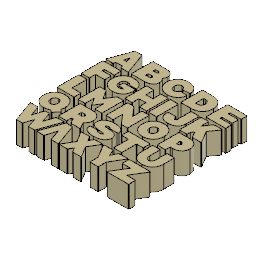
AlphaBlocks (Autodesk Fusion 360 design; units mm, degrees)
Autodesk Fusion 360 part; units mm, degrees
sketch "Sketch1" plane through (0, 0, 0) normal (0, 1, 0) x (1, 0, 0)
  arc A0 (47.4557, -43.7833) -> (46.9512, -43.2752) centre (47.4934, -43.2413) cw
  line L0 (46.9512, -43.2752) -> (46.9512, -18.8912)
  arc A1 (46.9512, -18.8912) -> (47.4557, -18.3833) centre (47.4934, -18.9252) cw
  line L1 (47.4557, -18.3833) -> (62.4769, -18.3833)
  spline S0 degree 3 poles (62.4769, -18.3833) (68.3824, -18.3833) (71.5045, -21.6429) (71.5045, -25.5799) knots 0 0 0 0 1 1 1 1
  arc A2 (71.5045, -25.5799) -> (69.5643, -30.1096) centre (65.5084, -25.6919) cw
  line L2 (69.5643, -30.1096) -> (69.5643, -30.1519)
  arc A3 (69.5643, -30.1519) -> (72.3512, -35.8669) centre (65.3567, -35.7408) cw
  spline S1 degree 3 poles (72.3512, -35.8669) (72.3512, -40.7353) (68.7211, -43.7833) (62.3923, -43.7833) knots 0 0 0 0 1 1 1 1
  line L3 (62.3923, -43.7833) -> (47.4557, -43.7833)
  line L4 (56.5679, -27.9083) -> (60.198, -27.9083)
  spline S2 degree 3 poles (60.198, -27.9083) (61.4645, -27.9083) (61.8843, -27.3579) (61.8843, -26.6383) knots 0 0 0 0 1 1 1 1
  spline S3 degree 3 poles (61.8843, -26.6383) (61.8843, -25.9186) (61.3798, -25.3683) (59.9863, -25.3683) knots 0 0 0 0 1 1 1 1
  line L5 (59.9863, -25.3683) -> (56.5679, -25.3683)
  line L6 (56.5679, -25.3683) -> (56.5679, -27.9083)
  line L7 (56.5679, -36.5866) -> (60.4943, -36.5866)
  spline S4 degree 3 poles (60.4943, -36.5866) (62.0536, -36.5866) (62.7309, -36.0786) (62.7309, -35.1472) knots 0 0 0 0 1 1 1 1
  spline S5 degree 3 poles (62.7309, -35.1472) (62.7309, -34.2159) (62.0536, -33.6232) (60.4943, -33.6232) knots 0 0 0 0 1 1 1 1
  line L8 (60.4943, -33.6232) -> (56.5679, -33.6232)
  line L9 (56.5679, -33.6232) -> (56.5679, -36.5866)
  spline S6 degree 3 poles (93.0698, -29.651) (92.7171, -29.651) (92.4913, -29.404) (92.3643, -28.9948) knots 0 0 0 0 1 1 1 1
  spline S7 degree 3 poles (92.3643, -28.9948) (91.8245, -27.111) (90.5545, -26.1726) (88.6636, -26.1726) knots 0 0 0 0 1 1 1 1
  spline S8 degree 3 poles (88.6636, -26.1726) (86.5823, -26.1726) (84.5397, -27.9753) (84.5397, -31.0868) knots 0 0 0 0 1 1 1 1
  spline S9 degree 3 poles (84.5397, -31.0868) (84.5397, -34.1171) (86.4694, -35.9622) (88.6636, -35.9622) knots 0 0 0 0 1 1 1 1
  spline S10 degree 3 poles (88.6636, -35.9622) (90.4275, -35.9622) (91.7469, -35.1014) (92.3643, -33.3798) knots 0 0 0 0 1 1 1 1
  arc A4 (92.3643, -33.3798) -> (93.1757, -32.7272) centre (93.1658, -33.5456) cw
  line L10 (93.1757, -32.7272) -> (100.4217, -32.7272)
  arc A5 (100.4217, -32.7272) -> (101.152, -33.4645) centre (100.3801, -33.4987) cw
  spline S11 degree 3 poles (101.152, -33.4645) (101.152, -39.5676) (95.7192, -43.7868) (88.6636, -43.7868) knots 0 0 0 0 1 1 1 1
  spline S12 degree 3 poles (88.6636, -43.7868) (81.4564, -43.7868) (75.752, -38.6256) (75.752, -31.0868) knots 0 0 0 0 1 1 1 1
  spline S13 degree 3 poles (75.752, -31.0868) (75.752, -23.5479) (81.4564, -18.3868) (88.6636, -18.3868) knots 0 0 0 0 1 1 1 1
  spline S14 degree 3 poles (88.6636, -18.3868) (95.9873, -18.3868) (101.152, -23.0576) (101.152, -28.8325) knots 0 0 0 0 1 1 1 1
  spline S15 degree 3 poles (101.152, -28.8325) (101.152, -29.2841) (100.9227, -29.6545) (100.4958, -29.6545) knots 0 0 0 0 1 1 1 1
  line L11 (100.4958, -29.6545) -> (93.0698, -29.651)
  arc A6 (105.0643, -43.7833) -> (104.5774, -43.2752) centre (105.113, -43.2492) cw
  line L12 (104.5774, -43.2752) -> (104.5774, -18.8912)
  arc A7 (104.5774, -18.8912) -> (105.0643, -18.3833) centre (105.113, -18.9173) cw
  line L13 (105.0643, -18.3833) -> (115.951, -18.3833)
  spline S16 degree 3 poles (115.951, -18.3833) (124.2695, -18.3833) (129.9774, -23.3786) (129.9774, -31.0833) knots 0 0 0 0 1 1 1 1
  spline S17 degree 3 poles (129.9774, -31.0833) (129.9774, -38.6609) (125.1656, -43.7833) (116.0321, -43.7833) knots 0 0 0 0 1 1 1 1
  line L14 (116.0321, -43.7833) -> (105.0643, -43.7833)
  line L15 (113.8837, -26.4266) -> (113.8837, -35.7399)
  line L16 (113.8837, -35.7399) -> (116.0004, -35.7399)
  spline S18 degree 3 poles (116.0004, -35.7399) (119.1401, -35.7399) (120.6888, -33.976) (120.6888, -31.0833) knots 0 0 0 0 1 1 1 1
  spline S19 degree 3 poles (120.6888, -31.0833) (120.6888, -28.1199) (118.8544, -26.4266) (115.9581, -26.4266) knots 0 0 0 0 1 1 1 1
  line L17 (115.9581, -26.4266) -> (113.8837, -26.4266)
  line L18 (143.5806, -34.6816) -> (143.5806, -36.5866)
  line L19 (143.5806, -36.5866) -> (156.3088, -36.5866)
  arc A8 (156.3088, -36.5866) -> (156.9014, -37.1792) centre (156.2038, -37.2843) cw
  line L20 (156.9014, -37.1792) -> (156.9014, -43.1765)
  arc A9 (156.9014, -43.1765) -> (156.3088, -43.7691) centre (156.2038, -43.0714) cw
  line L21 (156.3088, -43.7691) -> (134.4083, -43.7691)
  arc A10 (134.4083, -43.7691) -> (133.8968, -43.2611) centre (134.4423, -43.2234) cw
  line L22 (133.8968, -43.2611) -> (133.8968, -18.8912)
  arc A11 (133.8968, -18.8912) -> (134.4083, -18.3833) centre (134.4423, -18.929) cw
  line L23 (134.4083, -18.3833) -> (156.2982, -18.3833)
  arc A12 (156.2982, -18.3833) -> (156.8909, -18.9759) centre (156.1932, -19.0809) cw
  line L24 (156.8909, -18.9759) -> (156.8909, -24.9731)
  arc A13 (156.8909, -24.9731) -> (156.2982, -25.5658) centre (156.1932, -24.8681) cw
  line L25 (156.2982, -25.5658) -> (143.5806, -25.5658)
  line L26 (143.5806, -25.5658) -> (143.5806, -27.4708)
  line L27 (143.5806, -27.4708) -> (155.0353, -27.4708)
  arc A14 (155.0353, -27.4708) -> (155.6279, -28.0635) centre (154.9302, -28.1685) cw
  line L28 (155.6279, -28.0635) -> (155.6279, -34.0607)
  arc A15 (155.6279, -34.0607) -> (155.0353, -34.6534) centre (154.9302, -33.9557) cw
  line L29 (155.0353, -34.6534) -> (143.5806, -34.6816)
  arc A16 (17.6389, -72.2207) -> (17.1309, -71.7127) centre (17.6764, -71.6751) cw
  line L30 (17.1309, -71.7127) -> (17.1309, -47.3287)
  arc A17 (17.1309, -47.3287) -> (17.6389, -46.8207) centre (17.6764, -47.3662) cw
  line L31 (17.6389, -46.8207) -> (37.8319, -46.8207)
  arc A18 (37.8319, -46.8207) -> (38.4281, -47.4133) centre (37.7305, -47.5189) cw
  line L32 (38.4281, -47.4133) -> (38.4281, -54.2713)
  arc A19 (38.4281, -54.2713) -> (37.8319, -54.864) centre (37.7305, -54.1658) cw
  line L33 (37.8319, -54.864) -> (26.8111, -54.864)
  line L34 (26.8111, -54.864) -> (26.8111, -57.404)
  line L35 (26.8111, -57.404) -> (36.9923, -57.404)
  arc A20 (36.9923, -57.404) -> (37.5849, -57.9967) centre (36.8873, -58.1017) cw
  line L36 (37.5849, -57.9967) -> (37.5849, -64.4313)
  arc A21 (37.5849, -64.4313) -> (36.9923, -65.024) centre (36.8873, -64.3263) cw
  line L37 (36.9923, -65.024) -> (26.8111, -65.024)
  line L38 (26.8111, -65.024) -> (26.8111, -71.7268)
  arc A22 (26.8111, -71.7268) -> (26.2996, -72.2348) centre (26.2656, -71.689) cw
  line L39 (26.2996, -72.2348) -> (17.6389, -72.2207)
  arc A23 (83.4743, -119.9444) -> (84.7619, -120.6817) centre (83.5073, -121.3799) cw
  spline S20 degree 3 poles (84.7619, -120.6817) (85.217, -121.3379) (86.2154, -121.8283) (88.2474, -121.8283) knots 0 0 0 0 1 1 1 1
  spline S21 degree 3 poles (88.2474, -121.8283) (90.4064, -121.8283) (91.1542, -121.1227) (91.1542, -120.5195) knots 0 0 0 0 1 1 1 1
  spline S22 degree 3 poles (91.1542, -120.5195) (91.1542, -120.0679) (90.738, -119.8139) (89.535, -119.6975) knots 0 0 0 0 1 1 1 1
  line L40 (89.535, -119.6975) -> (83.7247, -119.126)
  spline S23 degree 3 poles (83.7247, -119.126) (78.6201, -118.6321) (75.2157, -116.5049) (75.2157, -112.3245) knots 0 0 0 0 1 1 1 1
  spline S24 degree 3 poles (75.2157, -112.3245) (75.2157, -106.9975) (79.9465, -103.2298) (87.4607, -103.2298) knots 0 0 0 0 1 1 1 1
  spline S25 degree 3 poles (87.4607, -103.2298) (95.5534, -103.2298) (99.1623, -106.7576) (99.1623, -110.1125) knots 0 0 0 0 1 1 1 1
  arc A24 (99.1623, -110.1125) -> (98.044, -111.3402) centre (97.9705, -110.1501) cw
  line L41 (98.044, -111.3402) -> (90.6956, -111.3402)
  arc A25 (90.6956, -111.3402) -> (89.7431, -110.8922) centre (90.6223, -110.2597) cw
  spline S26 degree 3 poles (89.7431, -110.8922) (89.3692, -110.4406) (88.706, -109.9467) (87.4183, -109.9467) knots 0 0 0 0 1 1 1 1
  spline S27 degree 3 poles (87.4183, -109.9467) (85.3828, -109.9467) (84.6772, -110.7264) (84.6772, -111.3014) knots 0 0 0 0 1 1 1 1
  spline S28 degree 3 poles (84.6772, -111.3014) (84.6772, -111.6542) (85.0124, -111.9541) (86.0072, -112.0387) knots 0 0 0 0 1 1 1 1
  line L42 (86.0072, -112.0387) -> (91.694, -112.5714)
  spline S29 degree 3 poles (91.694, -112.5714) (98.1675, -113.1852) (100.6158, -116.011) (100.6158, -119.821) knots 0 0 0 0 1 1 1 1
  spline S30 degree 3 poles (100.6158, -119.821) (100.6158, -124.7387) (96.2166, -128.6404) (87.6688, -128.6404) knots 0 0 0 0 1 1 1 1
  spline S31 degree 3 poles (87.6688, -128.6404) (80.0735, -128.6404) (75.4239, -125.4019) (75.4239, -121.472) knots 0 0 0 0 1 1 1 1
  line L43 (75.4239, -121.472) -> (75.4239, -121.225)
  arc A26 (75.4239, -121.225) -> (76.6692, -119.955) centre (76.756, -121.2857) cw
  line L44 (76.6692, -119.955) -> (83.4743, -119.9444)
  line L45 (62.4628, -144.0956) -> (62.2476, -144.0956)
  line L46 (62.2476, -144.0956) -> (58.4306, -156.0336)
  spline S32 degree 3 poles (58.4306, -156.0336) (58.2542, -156.4993) (58.0778, -156.5839) (57.6474, -156.5839) knots 0 0 0 0 1 1 1 1
  line L47 (57.6474, -156.5839) -> (49.9428, -156.5839)
  arc A27 (49.9428, -156.5839) -> (49.657, -156.2876) centre (49.9313, -156.309) cw
  arc A28 (49.657, -156.2876) -> (49.9075, -155.4833) centre (53.0992, -156.9184) cw
  line L48 (49.9075, -155.4833) -> (58.5611, -131.5191)
  arc A29 (58.5611, -131.5191) -> (59.0374, -131.1839) centre (59.0388, -131.6919) cw
  line L49 (59.0374, -131.1839) -> (65.6731, -131.1839)
  arc A30 (65.6731, -131.1839) -> (66.1529, -131.5191) centre (65.6727, -131.6955) cw
  line L50 (66.1529, -131.5191) -> (74.8065, -155.4833)
  arc A31 (74.8065, -155.4833) -> (75.057, -156.2876) centre (71.6148, -156.9184) cw
  arc A32 (75.057, -156.2876) -> (74.7713, -156.5839) centre (74.7827, -156.309) cw
  line L51 (74.7713, -156.5839) -> (67.0666, -156.5839)
  spline S33 degree 3 poles (67.0666, -156.5839) (66.6362, -156.5839) (66.4598, -156.4993) (66.2799, -156.0336) knots 0 0 0 0 1 1 1 1
  line L52 (66.2799, -156.0336) -> (62.4628, -144.0956)
  spline S34 degree 3 poles (65.8812, -59.9299) (65.8812, -66.6327) (61.8137, -72.2207) (53.3471, -72.2207) knots 0 0 0 0 1 1 1 1
  spline S35 degree 3 poles (53.3471, -72.2207) (45.8964, -72.2207) (40.4812, -66.9749) (40.4812, -59.5207) knots 0 0 0 0 1 1 1 1
  spline S36 degree 3 poles (40.4812, -59.5207) (40.4812, -52.0665) (45.8964, -46.8207) (53.3471, -46.8207) knots 0 0 0 0 1 1 1 1
  spline S37 degree 3 poles (53.3471, -46.8207) (61.3763, -46.8207) (65.1545, -51.9818) (65.1545, -55.4214) knots 0 0 0 0 1 1 1 1
  arc A33 (65.1545, -55.4214) -> (64.4666, -56.0388) centre (64.5443, -55.4334) cw
  line L53 (64.4666, -56.0388) -> (57.8167, -56.0388)
  arc A34 (57.8167, -56.0388) -> (56.9807, -55.5449) centre (57.8648, -55.0027) cw
  spline S38 degree 3 poles (56.9807, -55.5449) (56.4727, -54.8393) (55.5272, -54.1937) (53.5623, -54.1937) knots 0 0 0 0 1 1 1 1
  spline S39 degree 3 poles (53.5623, -54.1937) (50.74, -54.1937) (48.768, -56.4056) (48.768, -59.5207) knots 0 0 0 0 1 1 1 1
  spline S40 degree 3 poles (48.768, -59.5207) (48.768, -63.1649) (51.0928, -64.8441) (53.7069, -64.8441) knots 0 0 0 0 1 1 1 1
  spline S41 degree 3 poles (53.7069, -64.8441) (55.8871, -64.8441) (57.1571, -64.1068) (57.5874, -63.246) knots 0 0 0 0 1 1 1 1
  line L54 (57.5874, -63.246) -> (57.5874, -63.1649)
  line L55 (57.5874, -63.1649) -> (52.1123, -63.1649)
  arc A35 (52.1123, -63.1649) -> (51.6008, -62.5934) centre (52.2598, -62.5182) cw
  line L56 (51.6008, -62.5934) -> (51.6008, -57.7991)
  arc A36 (51.6008, -57.7991) -> (52.1123, -57.2241) centre (52.2602, -57.8706) cw
  line L57 (52.1123, -57.2241) -> (65.3732, -57.2241)
  arc A37 (65.3732, -57.2241) -> (65.8812, -57.7321) centre (65.3732, -57.7321) cw
  line L58 (65.8812, -57.7321) -> (65.8812, -59.9299)
  arc A38 (93.3485, -71.7127) -> (92.8934, -72.2207) centre (92.83, -71.706) cw
  line L59 (92.8934, -72.2207) -> (85.1606, -72.2207)
  arc A39 (85.1606, -72.2207) -> (84.7055, -71.7127) centre (85.224, -71.706) cw
  line L60 (84.7055, -71.7127) -> (84.7055, -64.3043)
  line L61 (84.7055, -64.3043) -> (76.5916, -64.3043)
  line L62 (76.5916, -64.3043) -> (76.5916, -71.7127)
  arc A40 (76.5916, -71.7127) -> (76.1365, -72.2207) centre (76.073, -71.706) cw
  line L63 (76.1365, -72.2207) -> (68.4036, -72.2207)
  arc A41 (68.4036, -72.2207) -> (67.9485, -71.7127) centre (68.4671, -71.706) cw
  line L64 (67.9485, -71.7127) -> (67.9485, -47.3287)
  arc A42 (67.9485, -47.3287) -> (68.4036, -46.8207) centre (68.4671, -47.3354) cw
  line L65 (68.4036, -46.8207) -> (76.1365, -46.8207)
  arc A43 (76.1365, -46.8207) -> (76.5916, -47.3287) centre (76.073, -47.3354) cw
  line L66 (76.5916, -47.3287) -> (76.5916, -56.261)
  line L67 (76.5916, -56.261) -> (84.7055, -56.261)
  line L68 (84.7055, -56.261) -> (84.7055, -47.3287)
  arc A44 (84.7055, -47.3287) -> (85.1605, -46.8207) centre (85.224, -47.3354) cw
  line L69 (85.1605, -46.8207) -> (92.8934, -46.8207)
  arc A45 (92.8934, -46.8207) -> (93.3485, -47.3287) centre (92.83, -47.3354) cw
  line L70 (93.3485, -47.3287) -> (93.3485, -71.7127)
  arc A46 (105.0854, -71.7656) -> (104.5774, -72.2736) centre (104.5399, -71.7281) cw
  line L71 (104.5774, -72.2736) -> (95.9238, -72.2736)
  arc A47 (95.9238, -72.2736) -> (95.4158, -71.7656) centre (95.9613, -71.7281) cw
  line L72 (95.4158, -71.7656) -> (95.4158, -47.3287)
  arc A48 (95.4158, -47.3287) -> (95.9238, -46.8207) centre (95.9613, -47.3662) cw
  line L73 (95.9238, -46.8207) -> (104.5774, -46.8207)
  arc A49 (104.5774, -46.8207) -> (105.0854, -47.3287) centre (104.5399, -47.3662) cw
  line L74 (105.0854, -47.3287) -> (105.0854, -71.7656)
  spline S42 degree 3 poles (116.8259, -62.5581) (116.8259, -63.7258) (117.4186, -64.322) (118.2687, -64.322) knots 0 0 0 0 1 1 1 1
  spline S43 degree 3 poles (118.2687, -64.322) (119.1189, -64.322) (119.7539, -63.7822) (119.7539, -62.5581) knots 0 0 0 0 1 1 1 1
  line L75 (119.7539, -62.5581) -> (119.7539, -47.3181)
  arc A50 (119.7539, -47.3181) -> (120.2619, -46.8207) centre (120.2921, -47.3596) cw
  line L76 (120.2619, -46.8207) -> (128.9156, -46.8207)
  arc A51 (128.9156, -46.8207) -> (129.4236, -47.3181) centre (128.8854, -47.3596) cw
  line L77 (129.4236, -47.3181) -> (129.4236, -62.0607)
  spline S44 degree 3 poles (129.4236, -62.0607) (129.4236, -67.8074) (125.9452, -72.2207) (117.9724, -72.2207) knots 0 0 0 0 1 1 1 1
  spline S45 degree 3 poles (117.9724, -72.2207) (110.0808, -72.2207) (107.1527, -67.8074) (107.1527, -63.4753) knots 0 0 0 0 1 1 1 1
  line L78 (107.1527, -63.4753) -> (107.1527, -61.8102)
  arc A52 (107.1527, -61.8102) -> (108.0876, -60.893) centre (108.177, -61.9192) cw
  line L79 (108.0876, -60.893) -> (116.2297, -60.893)
  arc A53 (116.2297, -60.893) -> (116.8259, -61.4751) centre (116.13, -61.5915) cw
  line L80 (116.8259, -61.4751) -> (116.8259, -62.5581)
  line L81 (140.3209, -55.5413) -> (140.4338, -55.5413)
  line L82 (140.4338, -55.5413) -> (146.1276, -47.4274)
  arc A54 (146.1276, -47.4274) -> (147.2107, -46.8348) centre (147.1942, -48.0906) cw
  line L83 (147.2107, -46.8348) -> (155.8078, -46.8348)
  arc A55 (155.8078, -46.8348) -> (156.3088, -47.3428) centre (155.8375, -47.3066) cw
  spline S46 degree 3 poles (156.3088, -47.3428) (156.3088, -47.4698) (156.27, -47.5968) (156.0019, -47.9778) knots 0 0 0 0 1 1 1 1
  line L84 (156.0019, -47.9778) -> (148.6817, -58.0955)
  line L85 (148.6817, -58.0955) -> (156.6969, -71.4305)
  spline S47 degree 3 poles (156.6969, -71.4305) (156.8521, -71.6845) (156.8909, -71.7832) (156.8909, -71.8961) knots 0 0 0 0 1 1 1 1
  arc A56 (156.8909, -71.8961) -> (156.5381, -72.2489) centre (156.5638, -71.9218) cw
  line L86 (156.5381, -72.2489) -> (147.2106, -72.2489)
  arc A57 (147.2106, -72.2489) -> (146.3604, -71.7832) centre (147.1576, -71.3367) cw
  line L87 (146.3604, -71.7832) -> (142.5222, -65.3627)
  line L88 (142.5222, -65.3627) -> (140.3174, -68.3683)
  line L89 (140.3174, -68.3683) -> (140.3174, -71.7127)
  arc A58 (140.3174, -71.7127) -> (139.8517, -72.2207) centre (139.7919, -71.6984) cw
  line L90 (139.8517, -72.2207) -> (131.9565, -72.2207)
  arc A59 (131.9565, -72.2207) -> (131.4909, -71.7127) centre (132.0163, -71.6984) cw
  line L91 (131.4909, -71.7127) -> (131.4909, -47.3287)
  arc A60 (131.4909, -47.3287) -> (131.9565, -46.8207) centre (132.0163, -47.3429) cw
  line L92 (131.9565, -46.8207) -> (139.8552, -46.8207)
  arc A61 (139.8552, -46.8207) -> (140.3209, -47.3287) centre (139.7954, -47.3429) cw
  line L93 (140.3209, -47.3287) -> (140.3209, -55.5413)
  line L94 (26.8111, -92.329) -> (36.5689, -92.329)
  arc A62 (36.5689, -92.329) -> (37.1616, -92.9217) centre (36.4639, -93.0267) cw
  line L95 (37.1616, -92.9217) -> (37.1616, -99.7797)
  arc A63 (37.1616, -99.7797) -> (36.5689, -100.3723) centre (36.4639, -99.6746) cw
  line L96 (36.5689, -100.3723) -> (17.6389, -100.3723)
  arc A64 (17.6389, -100.3723) -> (17.1309, -99.8643) centre (17.6764, -99.8268) cw
  line L97 (17.1309, -99.8643) -> (17.1309, -75.4944)
  arc A65 (17.1309, -75.4944) -> (17.6389, -74.9723) centre (17.6772, -75.5178) cw
  line L98 (17.6389, -74.9723) -> (26.2819, -74.9723)
  arc A66 (26.2819, -74.9723) -> (26.8111, -75.4944) centre (26.2649, -75.5189) cw
  line L99 (26.8111, -75.4944) -> (26.8111, -92.329)
  arc A67 (69.1233, -74.9723) -> (69.5678, -75.4944) centre (69.0529, -75.4826) cw
  line L100 (69.5678, -75.4944) -> (69.5678, -99.8784)
  arc A68 (69.5678, -99.8784) -> (69.1233, -100.3864) centre (69.0527, -99.8762) cw
  line L101 (69.1233, -100.3864) -> (61.6056, -100.3864)
  arc A69 (61.6056, -100.3864) -> (61.1611, -99.8784) centre (61.6761, -99.8762) cw
  line L102 (61.1611, -99.8784) -> (61.1611, -89.7184)
  line L103 (61.1611, -89.7184) -> (61.087, -89.7184)
  line L104 (61.087, -89.7184) -> (55.5978, -98.425)
  line L105 (55.5978, -98.425) -> (50.1403, -89.7043)
  line L106 (50.1403, -89.7043) -> (50.0309, -89.7043)
  line L107 (50.0309, -89.7043) -> (50.0309, -99.8643)
  arc A70 (50.0309, -99.8643) -> (49.5864, -100.3723) centre (49.5159, -99.8621) cw
  line L108 (49.5864, -100.3723) -> (42.0687, -100.3723)
  arc A71 (42.0687, -100.3723) -> (41.6278, -99.8643) centre (42.1393, -99.8657) cw
  line L109 (41.6278, -99.8643) -> (41.6278, -75.4944)
  arc A72 (41.6278, -75.4944) -> (42.0687, -74.9864) centre (42.1393, -75.4931) cw
  line L110 (42.0687, -74.9864) -> (48.6304, -74.9864)
  arc A73 (48.6304, -74.9864) -> (49.336, -75.4098) centre (48.6234, -75.7978) cw
  line L111 (49.336, -75.4098) -> (55.566, -84.9348)
  line L112 (55.566, -84.9348) -> (55.6401, -84.9348)
  line L113 (55.6401, -84.9348) -> (61.8702, -75.4098)
  arc A74 (61.8702, -75.4098) -> (62.5757, -74.9864) centre (62.5828, -75.7978) cw
  line L114 (62.5757, -74.9864) -> (69.1233, -74.9723)
  line L115 (82.8428, -89.6056) -> (82.6911, -89.6056)
  line L116 (82.6911, -89.6056) -> (82.6911, -99.8361)
  arc A75 (82.6911, -99.8361) -> (82.236, -100.3441) centre (82.1726, -99.8294) cw
  line L117 (82.236, -100.3441) -> (74.5031, -100.3441)
  arc A76 (74.5031, -100.3441) -> (74.0481, -99.8361) centre (74.5701, -99.8263) cw
  line L118 (74.0481, -99.8361) -> (74.0481, -75.4944)
  arc A77 (74.0481, -75.4944) -> (74.5031, -74.9864) centre (74.5701, -75.5042) cw
  line L119 (74.5031, -74.9864) -> (81.0966, -74.9864)
  arc A78 (81.0966, -74.9864) -> (81.4917, -75.1417) centre (81.1268, -75.49) cw
  line L120 (81.4917, -75.1417) -> (90.7062, -85.725)
  line L121 (90.7062, -85.725) -> (90.8191, -85.725)
  line L122 (90.8191, -85.725) -> (90.8191, -75.4944)
  arc A79 (90.8191, -75.4944) -> (91.2742, -74.9864) centre (91.3377, -75.5011) cw
  line L123 (91.2742, -74.9864) -> (99.0071, -74.9864)
  arc A80 (99.0071, -74.9864) -> (99.4481, -75.4944) centre (98.9295, -75.4992) cw
  line L124 (99.4481, -75.4944) -> (99.4481, -99.8784)
  arc A81 (99.4481, -99.8784) -> (98.993, -100.3864) centre (98.9295, -99.8718) cw
  line L125 (98.993, -100.3864) -> (92.4031, -100.3864)
  arc A82 (92.4031, -100.3864) -> (92.0186, -100.2101) centre (92.4066, -99.8714) cw
  line L126 (92.0186, -100.2101) -> (82.8428, -89.6056)
  arc A83 (134.3237, -100.3723) -> (133.8121, -99.8643) centre (134.3576, -99.8266) cw
  line L127 (133.8121, -99.8643) -> (133.8121, -75.4944)
  arc A84 (133.8121, -75.4944) -> (134.3237, -74.9864) centre (134.3576, -75.5322) cw
  line L128 (134.3237, -74.9864) -> (145.9477, -74.9864)
  spline S48 degree 3 poles (145.9477, -74.9864) (152.4353, -74.9864) (156.8838, -79.1774) (156.8838, -85.1464) knots 0 0 0 0 1 1 1 1
  spline S49 degree 3 poles (156.8838, -85.1464) (156.8838, -91.3271) (152.0896, -94.8831) (145.9477, -94.8831) knots 0 0 0 0 1 1 1 1
  line L129 (145.9477, -94.8831) -> (143.4783, -94.8831)
  line L130 (143.4783, -94.8831) -> (143.4783, -99.8784)
  arc A85 (143.4783, -99.8784) -> (142.9703, -100.3864) centre (142.9327, -99.8409) cw
  line L131 (142.9703, -100.3864) -> (134.3237, -100.3723)
  line L132 (143.4959, -83.0157) -> (143.4959, -87.6723)
  line L133 (143.4959, -87.6723) -> (144.8118, -87.6723)
  arc A86 (147.2283, -85.344) -> (144.8118, -87.6723) centre (144.9609, -85.4089) cw
  spline S50 degree 3 poles (147.2283, -85.344) (147.2283, -84.074) (146.424, -83.0157) (144.8118, -83.0157) knots 0 0 0 0 1 1 1 1
  line L134 (144.8118, -83.0157) -> (143.4959, -83.0157)
  arc A87 (47.0782, -103.7414) -> (47.5897, -103.2334) centre (47.627, -103.7824) cw
  line L135 (47.5897, -103.2334) -> (61.2881, -103.2334)
  spline S51 degree 3 poles (61.2881, -103.2334) (67.7968, -103.2334) (72.2665, -107.3397) (72.2665, -113.1817) knots 0 0 0 0 1 1 1 1
  arc A88 (72.2665, -113.1817) -> (68.1814, -120.7594) centre (63.4161, -113.3004) cw
  line L136 (68.1814, -120.7594) -> (68.1814, -120.844)
  line L137 (68.1814, -120.844) -> (72.2242, -127.6597)
  arc A89 (72.2242, -127.6597) -> (72.4782, -128.2947) centre (71.1071, -128.4748) cw
  spline S52 degree 3 poles (72.4782, -128.2947) (72.4782, -128.464) (72.3512, -128.6475) (72.0549, -128.6475) knots 0 0 0 0 1 1 1 1
  line L138 (72.0549, -128.6475) -> (62.2688, -128.6475)
  arc A90 (62.2688, -128.6475) -> (61.6726, -128.3511) centre (62.2476, -127.9422) cw
  line L139 (61.6726, -128.3511) -> (58.3953, -122.7067)
  line L140 (58.3953, -122.7067) -> (56.7972, -122.7067)
  line L141 (56.7972, -122.7067) -> (56.7972, -128.1254)
  arc A91 (56.7972, -128.1254) -> (56.2857, -128.6334) centre (56.2517, -128.0876) cw
  line L142 (56.2857, -128.6334) -> (47.5897, -128.6334)
  arc A92 (47.5897, -128.6334) -> (47.0782, -128.1254) centre (47.627, -128.0843) cw
  line L143 (47.0782, -128.1254) -> (47.0782, -103.7414)
  line L144 (56.7972, -111.2767) -> (56.7972, -115.0867)
  line L145 (56.7972, -115.0867) -> (60.325, -115.0867)
  spline S53 degree 3 poles (60.325, -115.0867) (62.0254, -115.0867) (62.5792, -114.0707) (62.5792, -113.1817) knots 0 0 0 0 1 1 1 1
  spline S54 degree 3 poles (62.5792, -113.1817) (62.5792, -112.2927) (61.9831, -111.2767) (60.325, -111.2767) knots 0 0 0 0 1 1 1 1
  line L146 (60.325, -111.2767) -> (56.7972, -111.2767)
  arc A93 (103.9354, -111.2767) -> (103.3533, -110.684) centre (104.0513, -110.5807) cw
  line L147 (103.3533, -110.684) -> (103.3533, -103.826)
  arc A94 (103.3533, -103.826) -> (103.9354, -103.2334) centre (104.0513, -103.9293) cw
  line L148 (103.9354, -103.2334) -> (128.1712, -103.2334)
  arc A95 (128.1712, -103.2334) -> (128.7533, -103.826) centre (128.0554, -103.9293) cw
  line L149 (128.7533, -103.826) -> (128.7533, -110.684)
  arc A96 (128.7533, -110.684) -> (128.1712, -111.2767) centre (128.0554, -110.5807) cw
  line L150 (128.1712, -111.2767) -> (121.3097, -111.2767)
  arc A97 (120.8017, -111.7847) -> (121.3097, -111.2767) centre (121.3062, -111.7812) cw
  line L151 (120.8017, -111.7847) -> (120.8017, -128.1254)
  arc A98 (120.8017, -128.1254) -> (120.3007, -128.6334) centre (120.2595, -128.0917) cw
  line L152 (120.3007, -128.6334) -> (111.8059, -128.6334)
  arc A99 (111.8059, -128.6334) -> (111.3084, -128.1254) centre (111.8473, -128.0952) cw
  line L153 (111.3084, -128.1254) -> (111.3084, -111.7847)
  arc A100 (110.8004, -111.2767) -> (111.3084, -111.7847) centre (110.8004, -111.7847) cw
  line L154 (110.8004, -111.2767) -> (103.9354, -111.2767)
  arc A101 (148.0079, -103.7167) -> (148.4771, -103.2192) centre (148.5296, -103.7387) cw
  line L155 (148.4771, -103.2192) -> (156.4252, -103.2192)
  arc A102 (156.4252, -103.2192) -> (156.8909, -103.7167) centre (156.3726, -103.7352) cw
  line L156 (156.8909, -103.7167) -> (156.8909, -115.7111)
  spline S55 degree 3 poles (156.8909, -115.7111) (156.8909, -123.7897) (152.2165, -128.6192) (144.1909, -128.6192) knots 0 0 0 0 1 1 1 1
  spline S56 degree 3 poles (144.1909, -128.6192) (136.1652, -128.6192) (131.4909, -123.7897) (131.4909, -115.7111) knots 0 0 0 0 1 1 1 1
  line L157 (131.4909, -115.7111) -> (131.4909, -103.7167)
  arc A103 (131.4909, -103.7167) -> (131.96, -103.2192) centre (132.0125, -103.7387) cw
  line L158 (131.96, -103.2192) -> (139.9046, -103.2192)
  arc A104 (139.9046, -103.2192) -> (140.3738, -103.7167) centre (139.8521, -103.7387) cw
  line L159 (140.3738, -103.7167) -> (140.3738, -115.503)
  spline S57 degree 3 poles (140.3738, -115.503) (140.3738, -118.9179) (141.8131, -120.7064) (144.1908, -120.7064) knots 0 0 0 0 1 1 1 1
  spline S58 degree 3 poles (144.1908, -120.7064) (146.5686, -120.7064) (148.0079, -118.9179) (148.0079, -115.503) knots 0 0 0 0 1 1 1 1
  line L160 (148.0079, -115.503) -> (148.0079, -103.7167)
  line L161 (47.177, -156.5839) -> (40.6506, -156.5839)
  arc A105 (40.6506, -156.5839) -> (40.1673, -156.2312) centre (40.651, -156.0759) cw
  line L162 (40.1673, -156.2312) -> (36.8441, -146.05)
  line L163 (36.8441, -146.05) -> (36.7665, -146.05)
  line L164 (36.7665, -146.05) -> (33.4433, -156.2347)
  arc A106 (33.4433, -156.2347) -> (32.96, -156.5875) centre (32.9622, -156.083) cw
  line L165 (32.96, -156.5875) -> (26.4336, -156.5875)
  arc A107 (26.4336, -156.5875) -> (25.9539, -156.2523) centre (26.434, -156.0759) cw
  line L166 (25.9539, -156.2523) -> (17.2332, -131.9389)
  arc A108 (17.2332, -131.9389) -> (17.1203, -131.4732) centre (18.563, -131.37) cw
  arc A109 (17.1203, -131.4732) -> (17.4237, -131.1769) centre (17.4058, -131.4621) cw
  line L167 (17.4237, -131.1769) -> (25.5834, -131.1769)
  spline S59 degree 3 poles (25.5834, -131.1769) (26.0385, -131.1769) (26.2255, -131.2616) (26.416, -131.8119) knots 0 0 0 0 1 1 1 1
  line L168 (26.416, -131.8119) -> (30.2683, -142.9103)
  line L169 (30.2683, -142.9103) -> (30.3812, -142.9103)
  line L170 (30.3812, -142.9103) -> (34.1171, -131.5261)
  arc A110 (34.1171, -131.5261) -> (34.6004, -131.1734) centre (34.6034, -131.6849) cw
  line L171 (34.6004, -131.1734) -> (39.0102, -131.1734)
  arc A111 (39.0102, -131.1734) -> (39.4899, -131.5261) centre (39.0114, -131.6743) cw
  line L172 (39.4899, -131.5261) -> (43.2294, -142.9068)
  line L173 (43.2294, -142.9068) -> (43.3035, -142.9068)
  line L174 (43.3035, -142.9068) -> (47.184, -131.8154)
  arc A112 (47.184, -131.8154) -> (48.0166, -131.1804) centre (47.9678, -131.9797) cw
  line L175 (48.0166, -131.1804) -> (56.1763, -131.1804)
  arc A113 (56.1763, -131.1804) -> (56.4797, -131.4768) centre (56.1979, -131.4618) cw
  arc A114 (56.4797, -131.4768) -> (56.3668, -131.9424) centre (54.7492, -131.3037) cw
  line L176 (56.3668, -131.9424) -> (47.6462, -156.2453)
  arc A115 (47.6462, -156.2453) -> (47.177, -156.5839) centre (47.1647, -156.0726) cw
  line L177 (89.1434, -136.1722) -> (89.2175, -136.1722)
  line L178 (89.2175, -136.1722) -> (91.5176, -131.8119)
  spline S60 degree 3 poles (91.5176, -131.8119) (91.8104, -131.2616) (92.0291, -131.1769) (92.4701, -131.1769) knots 0 0 0 0 1 1 1 1
  line L179 (92.4701, -131.1769) -> (101.0955, -131.1769)
  arc A116 (101.0955, -131.1769) -> (101.3143, -131.4309) centre (101.0863, -131.406) cw
  arc A117 (101.3143, -131.4309) -> (101.1661, -131.8119) centre (100.5594, -131.3567) cw
  line L180 (101.1661, -131.8119) -> (93.8953, -143.8769)
  line L181 (93.8953, -143.8769) -> (101.3495, -155.9842)
  arc A118 (101.3495, -155.9842) -> (101.4977, -156.337) centre (100.8415, -156.4051) cw
  arc A119 (101.4977, -156.337) -> (101.2755, -156.591) centre (101.2659, -156.3584) cw
  line L182 (101.2755, -156.591) -> (92.3219, -156.591)
  arc A120 (92.3219, -156.591) -> (91.4471, -156.083) centre (92.232, -155.7385) cw
  line L183 (91.4471, -156.083) -> (88.5966, -151.4687)
  line L184 (88.5966, -151.4687) -> (88.5225, -151.4687)
  line L185 (88.5225, -151.4687) -> (85.8908, -156.083)
  arc A121 (85.8908, -156.083) -> (85.0124, -156.591) centre (85.1211, -155.7656) cw
  line L186 (85.0124, -156.591) -> (76.3164, -156.591)
  arc A122 (76.3164, -156.591) -> (76.0977, -156.337) centre (76.3256, -156.3619) cw
  arc A123 (76.0977, -156.337) -> (76.2423, -155.956) centre (76.8393, -156.4006) cw
  line L187 (76.2423, -155.956) -> (83.6507, -143.51)
  line L188 (83.6507, -143.51) -> (76.4505, -131.7837)
  arc A124 (76.4505, -131.7837) -> (76.3058, -131.4309) centre (77.2183, -131.2628) cw
  arc A125 (76.3058, -131.4309) -> (76.5246, -131.1769) centre (76.5338, -131.406) cw
  line L189 (76.5246, -131.1769) -> (85.5133, -131.1769)
  spline S61 degree 3 poles (85.5133, -131.1769) (85.9543, -131.1769) (86.1377, -131.2616) (86.4658, -131.8119) knots 0 0 0 0 1 1 1 1
  line L190 (86.4658, -131.8119) -> (89.1434, -136.1722)
  arc A126 (121.4579, -156.0759) -> (120.9463, -156.5839) centre (120.9124, -156.0382) cw
  line L191 (120.9463, -156.5839) -> (112.2927, -156.5839)
  arc A127 (112.2927, -156.5839) -> (111.7847, -156.0759) centre (112.3302, -156.0384) cw
  line L192 (111.7847, -156.0759) -> (111.7847, -147.2565)
  line L193 (111.7847, -147.2565) -> (102.6583, -131.7766)
  arc A128 (102.6583, -131.7766) -> (102.5313, -131.4238) centre (103.3717, -131.3206) cw
  arc A129 (102.5313, -131.4238) -> (102.8312, -131.1698) centre (102.8154, -131.4551) cw
  line L194 (102.8312, -131.1698) -> (112.4585, -131.1698)
  spline S62 degree 3 poles (112.4585, -131.1698) (112.97, -131.1698) (113.2664, -131.2545) (113.478, -131.6778) knots 0 0 0 0 1 1 1 1
  line L195 (113.478, -131.6778) -> (116.5331, -138.5782)
  line L196 (116.5331, -138.5782) -> (116.7024, -138.5782)
  line L197 (116.7024, -138.5782) -> (119.7575, -131.6778)
  spline S63 degree 3 poles (119.7575, -131.6778) (119.9692, -131.2545) (120.2655, -131.1698) (120.7735, -131.1698) knots 0 0 0 0 1 1 1 1
  line L198 (120.7735, -131.1698) -> (130.4043, -131.1698)
  arc A130 (130.4043, -131.1698) -> (130.7007, -131.4238) centre (130.4198, -131.4516) cw
  spline S64 degree 3 poles (130.7007, -131.4238) (130.7007, -131.5085) (130.7007, -131.5508) (130.5737, -131.7766) knots 0 0 0 0 1 1 1 1
  line L199 (130.5737, -131.7766) -> (121.4544, -147.2706)
  line L200 (121.4544, -147.2706) -> (121.4579, -156.0759)
  line L201 (141.6367, -139.3472) -> (141.6367, -139.2202)
  line L202 (141.6367, -139.2202) -> (132.4645, -139.2202)
  arc A131 (132.4645, -139.2202) -> (131.9036, -138.6276) centre (132.4856, -138.6385) cw
  line L203 (131.9036, -138.6276) -> (131.9036, -131.7766)
  arc A132 (131.9036, -131.7766) -> (132.4645, -131.1839) centre (132.4856, -131.7657) cw
  line L204 (132.4645, -131.1839) -> (156.4111, -131.1839)
  arc A133 (156.4111, -131.1839) -> (156.8133, -131.9671) centre (156.3866, -131.6914) cw
  line L205 (156.8133, -131.9671) -> (146.5545, -148.4559)
  line L206 (146.5545, -148.4559) -> (146.5545, -148.5406)
  line L207 (146.5545, -148.5406) -> (156.3335, -148.5406)
  arc A134 (156.3335, -148.5406) -> (156.8979, -149.1333) centre (156.3159, -149.1224) cw
  line L208 (156.8979, -149.1333) -> (156.8979, -155.9913)
  arc A135 (156.8979, -155.9913) -> (156.3335, -156.5839) centre (156.3159, -156.0021) cw
  line L209 (156.3335, -156.5839) -> (131.9918, -156.5839)
  arc A136 (131.9918, -156.5839) -> (131.5861, -155.8043) centre (132.0151, -156.0765) cw
  line L210 (131.5861, -155.8043) -> (141.6367, -139.3472)
  line L211 (34.103, -41.0316) -> (26.5536, -41.0316)
  line L212 (26.5536, -41.0316) -> (25.848, -43.2329)
  arc A137 (25.848, -43.2329) -> (25.1142, -43.7832) centre (25.2085, -43.1446) cw
  line L213 (25.1142, -43.7832) -> (17.399, -43.7832)
  arc A138 (17.399, -43.7832) -> (17.1203, -43.4869) centre (17.3947, -43.5081) cw
  arc A139 (17.1203, -43.4869) -> (17.2614, -42.9789) centre (19.1116, -43.7665) cw
  line L214 (17.2614, -42.9789) -> (26.2043, -18.3833)
  line L215 (26.2043, -18.3833) -> (34.4523, -18.3833)
  line L216 (34.4523, -18.3833) -> (43.3917, -42.9789)
  arc A140 (43.3917, -42.9789) -> (43.5328, -43.4869) centre (41.9091, -43.6643) cw
  arc A141 (43.5328, -43.4869) -> (43.2541, -43.7833) centre (43.2584, -43.5081) cw
  line L217 (43.2541, -43.7833) -> (35.5353, -43.7833)
  arc A142 (35.5353, -43.7833) -> (34.8015, -43.2329) centre (35.441, -43.1446) cw
  line L218 (34.8015, -43.2329) -> (34.103, -41.0316)
  line L219 (28.7549, -34.0466) -> (31.8664, -34.0466)
  line L220 (31.8664, -34.0466) -> (30.4553, -28.5433)
  line L221 (30.4553, -28.5433) -> (30.1731, -28.5433)
  line L222 (30.1731, -28.5433) -> (28.7549, -34.0466)
  spline S65 degree 3 poles (129.3319, -87.6723) (129.3319, -95.6204) (123.4616, -100.3723) (116.6319, -100.3723) knots 0 0 0 0 1 1 1 1
  spline S66 degree 3 poles (116.6319, -100.3723) (109.8021, -100.3723) (103.9319, -95.6204) (103.9319, -87.6723) knots 0 0 0 0 1 1 1 1
  spline S67 degree 3 poles (103.9319, -87.6723) (103.9319, -79.7243) (109.8374, -74.9723) (116.6319, -74.9723) knots 0 0 0 0 1 1 1 1
  spline S68 degree 3 poles (116.6319, -74.9723) (123.4969, -74.9723) (129.3319, -79.7278) (129.3319, -87.6723) knots 0 0 0 0 1 1 1 1
  spline S69 degree 3 poles (112.3491, -87.7111) (112.3491, -90.745) (114.3776, -92.5865) (116.6319, -92.5865) knots 0 0 0 0 1 1 1 1
  spline S70 degree 3 poles (116.6319, -92.5865) (118.8861, -92.5865) (120.9146, -90.745) (120.9146, -87.7111) knots 0 0 0 0 1 1 1 1
  spline S71 degree 3 poles (120.9146, -87.7111) (120.9146, -84.5573) (118.8826, -82.7723) (116.6319, -82.7723) knots 0 0 0 0 1 1 1 1
  spline S72 degree 3 poles (116.6319, -82.7723) (114.3811, -82.7723) (112.3491, -84.5573) (112.3491, -87.7111) knots 0 0 0 0 1 1 1 1
  line L223 (44.1572, -122.3363) -> (41.8183, -120.4066)
  arc A143 (42.5238, -115.9334) -> (41.8183, -120.4066) centre (28.4976, -116.0133) cw
  spline S73 degree 3 poles (42.5238, -115.9334) (42.5238, -107.9853) (36.6889, -103.2334) (29.8238, -103.2334) knots 0 0 0 0 1 1 1 1
  spline S74 degree 3 poles (29.8238, -103.2334) (23.0293, -103.2334) (17.1238, -107.9853) (17.1238, -115.9334) knots 0 0 0 0 1 1 1 1
  spline S75 degree 3 poles (17.1238, -115.9334) (17.1238, -123.8814) (23.0293, -128.6334) (29.8238, -128.6334) knots 0 0 0 0 1 1 1 1
  arc A144 (36.7665, -126.7566) -> (29.8238, -128.6334) centre (29.9423, -115.2918) cw
  line L224 (36.7665, -126.7566) -> (38.9925, -128.5946)
  arc A145 (39.6981, -128.524) -> (38.9925, -128.5946) centre (39.3091, -128.1973) cw
  line L225 (39.6981, -128.524) -> (44.2172, -123.0524)
  arc A146 (44.1572, -122.3363) -> (44.2172, -123.0524) centre (43.8293, -122.7243) cw
  spline S76 degree 3 poles (29.8203, -120.8511) (27.5696, -120.8511) (25.5376, -119.0061) (25.5376, -115.9757) knots 0 0 0 0 1 1 1 1
  spline S77 degree 3 poles (25.5376, -115.9757) (25.5376, -112.8183) (27.5696, -111.0156) (29.8203, -111.0156) knots 0 0 0 0 1 1 1 1
  spline S78 degree 3 poles (29.8203, -111.0156) (32.071, -111.0156) (34.103, -112.8183) (34.103, -115.9757) knots 0 0 0 0 1 1 1 1
  spline S79 degree 3 poles (34.103, -115.9757) (34.103, -119.0061) (32.071, -120.8511) (29.8203, -120.8511) knots 0 0 0 0 1 1 1 1
extrude "Extrude1" add sketch "Sketch1" along normal blind 25.4 makes body 1 at (95.8556, 0, 152.1507) makes body 2 at (47.0782, 8.4667, 119.9974) makes body 3 at (133.8121, 8.4667, 91.741) makes body 4 at (17.1309, 8.4667, 91.741) makes body 5 at (95.4158, 8.4667, 63.6199) makes body 6 at (104.5774, 8.4667, 35.1472) makes body 7 at (20.2424, 8.4667, 34.7804) makes body 8 at (133.8968, 8.4667, 35.1378) makes body 9 at (67.9485, 8.4667, 63.5847) makes body 10 at (69.5678, 8.4667, 83.6224) makes body 11 at (131.6622, 11.2889, 118.2815) makes body 12 at (42.3143, 14.1111, 113.4045) makes body 13 at (124.4941, 16.9333, 142.106) makes body 14 at (69.0374, 8.4667, 139.5071) makes body 15 at (86.4223, 0, 116.9541) makes body 16 at (129.1223, 14.1111, 85.1444) makes body 17 at (17.1309, 8.4667, 63.5847) makes body 18 at (120.4649, 11.2889, 72.0614) makes body 19 at (75.9575, 14.1111, 28.6657) makes body 20 at (46.9512, 8.4667, 35.1472) makes body 21 at (131.4909, 8.4667, 63.5847) makes body 22 at (50.9435, 11.2889, 47.0108) makes body 23 at (99.4481, 8.4667, 83.6224) makes body 24 at (112.014, 8.4667, 103.2334) makes body 25 at (23.047, 16.9333, 148.1478) makes body 26 at (148.2196, 8.4667, 156.5839)
